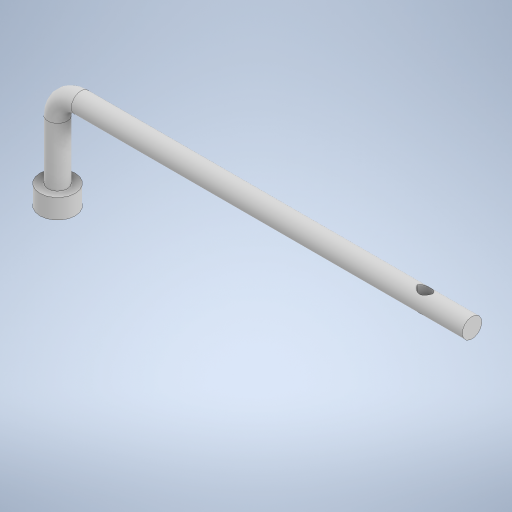
# Autodesk Inventor part: Chave
Saved by Autodesk Inventor 2024 (Build 280153000, 153)
## iProperties
Created: 2024-06-26
Part Number: Chave
Material: Generic
Document SubType Name: Modeling
Designer: Pedro
Density: 1 g/cm^3
Appearance: Default
Author: Pedro
Autodesk Inventor part; units mm, degrees
ref_plane "YZ Plane" through (0, 0, 0) normal (1, 0, 0) x (0, 1, 0)
ref_plane "XZ Plane" through (0, 0, 0) normal (0, 1, 0) x (-1, 0, 0)
ref_plane "XY Plane" through (0, 0, 0) normal (0, 0, 1) x (1, 0, 0)
sketch "Sketch1" plane through (0, 0, 0) normal (0, 1, 0) x (-1, 0, 0)
  arc A0 (-450, 0) -> (-430, 0) centre (-440, 3.6429) ccw
  arc A1 (-430, 0) -> (-450, 0) centre (-440, -3.6429) ccw
  constraints: 4 point on circle, 2 centre point
sketch "Sketch2" plane through (0, 0, 0) normal (1, 0, 0) x (0, 1, 0)
  circle A0 centre (0, 0) radius 12.5
  dimension "d8" = 25
  constraints: 1 centre point, 1 coincident
  measures "d8" diameter of A0
extrude "Extrusion1" add sketch "Sketch2" along normal blind 500
extrude "Extrusion2" cut sketch "Sketch1" along normal mid plane 25
sketch "Sketch3" plane through (0, 0, 0) normal (0, 0, 1) x (1, 0, 0)
  line L0 (0, -12.5) -> (0, 12.5) projected
  line L1 (0, -30) -> (-42.5, -30) construction
  line L2 (0, -30) -> (0, 12.5) construction
  line L3 (-17.5, -30) -> (-17.5, -105)
  line L4 (-17.5, -105) -> (-7.5, -105)
  line L5 (-7.5, -105) -> (-7.5, -130)
  line L6 (-7.5, -130) -> (-30, -130)
  line L7 (-30, -130) -> (-30, -30)
  line L8 (-17.5, -30) -> (-30, -30)
  point P0 (0, 0)
  point P1 (0, 0)
  dimension "d13" = 90
  dimension "d14" = 30
  dimension "d15" = 75
  dimension "d16" = 10
  dimension "d17" = 25
  dimension "d18" = 22.5
  constraints: 16 end point, 2 horizontal, 2 perpendicular, 2 vertical, 1 midpoint, 1 point on line
  measures "d13" angle of L2 L1
  measures "d14" distance of point (0, 0) L1.start
  measures "d15" distance of L3.start L3.end
  measures "d16" distance of L3.end L4.end
  measures "d17" distance of L4.end L5.end
  measures "d18" distance of L5.end L6.end
revolve "Revolution1" add sketch "Sketch3" angle 360 about axis through (-30, -130, 0) along (0, 1, 0)
sketch "Sketch5" plane through (0, 0, 0) normal (-1, 0, 0) x (0, 0, 1)
  circle A0 centre (0, 0) radius 12.5
  line L0 (12.5, -30) -> (-12.5, -30) projected
  line L1 (12.5, -30) -> (-12.5, -30)
  constraints: 2 end point, 1 centre point, 1 coincident, 1 collinear
revolve "Revolution2" add sketch "Sketch5" angle 90 about axis through (0, -30, 12.5) along (0, 0, 1)
sketch "Sketch6" plane through (-30, -130, 0) normal (0, -1, 0) x (1, 0, 0)
  line L0 (-10.5, -0.0258) -> (-5.25, 9.0675)
  line L1 (-5.25, 9.0675) -> (5.25, 9.0675)
  line L2 (5.25, 9.0675) -> (10.5, -0.0258)
  line L3 (10.5, -0.0258) -> (5.25, -9.119)
  line L4 (5.25, -9.119) -> (-5.25, -9.119)
  line L5 (-5.25, -9.119) -> (-10.5, -0.0258)
  circle A0 centre (0, 0) radius 22.5 projected
  point P0 (30, 0)
  point P1 (0, 9.0675)
  dimension "d24" = 120
  dimension "d25" = 21
  dimension "d26" = 120
  dimension "d27" = 120
  dimension "d28" = 0
  dimension "d29" = 120
  dimension "d30" = 0
  dimension "d31" = 10.5
  dimension "d32" = 10.5
  constraints: 12 end point, 1 horizontal, 1 midpoint, 1 parallel
  measures "d24" angle of L5 L0
  measures "d25" distance of L2.end L0.start
  measures "d26" angle of L1 L0
  measures "d27" angle of L2 L1
  measures "d28" vertical distance of L2.end L0.start
  measures "d29" angle of L3 L2
  measures "d30" horizontal distance of A0.centre point (0, 9.067)
  measures "d31" distance of L0.end L1.end
  measures "d32" distance of L3.end L4.end
extrude "Extrusion3" cut sketch "Sketch6" against normal blind 20 contours L0 L1 L2 L3 L4 L5
body "Solid1"
